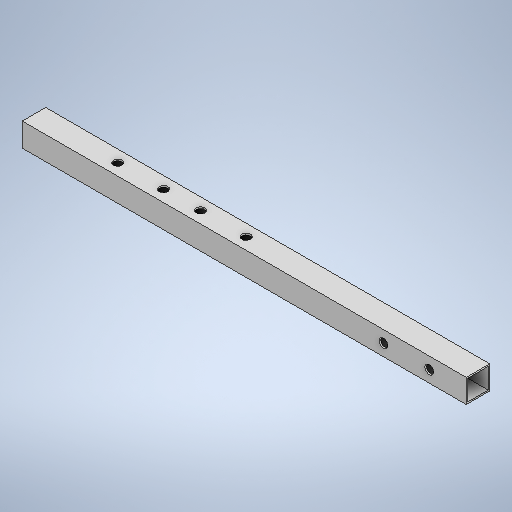
# Autodesk Inventor part: Base_Fija_Acero
Saved by Autodesk Inventor 2025.2 (Build 292293000, 293)
## iProperties
Created: 2025-05-30
Part Number: Base_Fija_Acero
Material: Generic
Document SubType Name: Modeling
Designer: USER
Density: 1 g/cm^3
Appearance: Default
Author: USER
Autodesk Inventor part; units mm, degrees
ref_plane "YZ Plane" through (0, 0, 0) normal (1, 0, 0) x (0, 1, 0)
ref_plane "XZ Plane" through (0, 0, 0) normal (0, 1, 0) x (-1, 0, 0)
ref_plane "XY Plane" through (0, 0, 0) normal (0, 0, 1) x (1, 0, 0)
sketch "Sketch1" plane through (0, 0, 0) normal (1, 0, 0) x (0, 1, 0)
  line L0 (0, 0) -> (31.75, 0)
  line L1 (31.75, 0) -> (31.75, -31.75)
  line L2 (31.75, -31.75) -> (0, -31.75)
  line L3 (0, -31.75) -> (0, 0)
  line L4 (29.75, -29.75) -> (29.75, -2)
  line L5 (29.75, -2) -> (2, -2)
  line L6 (2, -2) -> (2, -29.75)
  line L7 (2, -29.75) -> (29.75, -29.75)
  dimension "d0" = 31.75
  dimension "d1" = 31.75
  dimension "d2" = 2
  constraints: 16 end point, 4 parallel, 2 perpendicular, 1 horizontal, 3 other
  measures "d0" distance of L1.end L2.end
  measures "d1" distance of L0.end L1.end
  measures "d2" distance between parallel lines of L1 L4
extrude "Extrusion1" add sketch "Sketch1" along normal blind 600
sketch "Sketch2" plane through (0, 31.75, 0) normal (0, 1, 0) x (1, 0, 0)
  line L0 (0, 0) -> (600, 0) projected
  line L1 (600, 0) -> (400, 0)
  line L2 (0, 0) -> (400, 0)
  line L3 (0, 0) -> (400, 0)
  line L4 (0, 0) -> (200, 0)
  line L5 (0, 31.75) -> (0, 0) projected
  line L6 (0, 0) -> (600, 0) projected
  line L7 (600, 31.75) -> (600, 0) projected
  line L8 (0, 31.75) -> (600, 31.75) projected
  circle A0 centre (286.75, 15.875) radius 6
  circle A1 centre (113.25, 15.875) radius 6
  circle A2 centre (175, 15.875) radius 6
  circle A3 centre (225, 15.875) radius 6
  dimension "d5" = 200
  dimension "d6" = 200
  dimension "d7" = 12
  dimension "d8" = 86.75
  dimension "d9" = 12
  dimension "d10" = 86.75
  dimension "d11" = 12
  dimension "d12" = 61.75
  dimension "d13" = 12
  dimension "d14" = 61.75
  constraints: 8 end point, 4 centre point, 3 midpoint, 1 collinear, 1 point on line
  measures "d5" distance of L0.end L1.end
  measures "d6" distance of L0.start L4.end
  measures "d7" diameter of A0
  measures "d8" horizontal distance of A0.centre point (200, 0)
  measures "d9" diameter of A1
  measures "d10" horizontal distance of A1.centre point (200, 0)
  measures "d11" diameter of A2
  measures "d12" distance of A1.centre A2.centre
  measures "d13" diameter of A3
  measures "d14" distance of A3.centre A0.centre
extrude "Extrusion2" cut sketch "Sketch2" against normal through all contours A0 | A1 | A2 | A3
sketch "Sketch3" plane through (0, 0, -31.75) normal (0, 0, -1) x (-1, 0, 0)
  line L0 (-600, 0) -> (-550, 0)
  line L1 (0, 0) -> (-600, 0) projected
  line L2 (0, 0) -> (0, 31.75) projected
  line L3 (0, 31.75) -> (-600, 31.75) projected
  line L4 (-600, 0) -> (-600, 31.75) projected
  line L5 (0, 0) -> (-600, 0) projected
  circle A0 centre (-550, 15.875) radius 6
  circle A1 centre (-488.25, 15.875) radius 6
  dimension "d17" = 50
  dimension "d19" = 12
  dimension "d20" = 12
  dimension "d21" = 61.75
  constraints: 2 centre point, 2 end point, 1 point on line
  measures "d17" distance of L0.start L0.end
  measures "d19" diameter of A0
  measures "d20" diameter of A1
  measures "d21" distance of A0.centre A1.centre
extrude "Extrusion3" cut sketch "Sketch3" against normal through all contours A0 | A1
body "Solid1"
